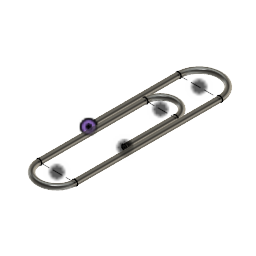
Day3Paperclip (Autodesk Fusion 360 design; units mm, degrees)
part number: 2025-11-19-20-14-40-836
Autodesk Fusion 360 part; units mm, degrees
sketch "Sweep" plane through (0, 0, 0) normal (0, 0, 1) x (1, 0, 0)
  line L0 (0, 0) -> (0, 16.25)
  line L1 (0, 16.25) -> (7.5, 16.25) construction
  line L2 (7.5, 16.25) -> (7.5, -10)
  line L3 (1, -10) -> (1, 9.25)
  line L4 (7.5, -10) -> (1, -10) construction
  line L5 (1, 9.25) -> (6.5, 9.25) construction
  line L6 (6.5, 9.25) -> (6.5, 0)
  arc A0 (7.5, 16.25) -> (0, 16.25) centre (3.75, 16.25) ccw
  arc A1 (6.5, 9.25) -> (1, 9.25) centre (3.75, 9.25) ccw
  arc A2 (1, -10) -> (7.5, -10) centre (4.25, -10) ccw
  dimension "d1" = 16.25
  dimension "d2" = 7.5
  dimension "d4" = 19.25
  dimension "d5" = 5.5
  dimension "d6" = 26.25
  dimension "d7" = 6.5
  dimension "d8" = 9.25
  constraint coincident L0.start origin
  constraint vertical L0
  constraint perpendicular L0 L1
  constraint perpendicular L1 L2
  constraint perpendicular L3 L4
  constraint perpendicular L3 L5
  constraint perpendicular L4 L6
  constraint vertical L3
  constraint tangent L0 A0
  constraint tangent L3 A1
  constraint tangent L3 A2
  measures "d1" distance of L0.start L0.end
  measures "d2" distance of L0.end L1.end
  measures "d4" distance of L3.start L3.end
  measures "d5" distance of L3.end L5.end
  measures "d6" distance of L1.end L2.end
  measures "d7" distance of L2.end L3.start
  measures "d8" distance of L5.end L6.end
sketch "Sketch2" plane through (0, 0, 0) normal (0, 1, 0) x (1, 0, 0)
  circle A0 centre (0, 0) radius 0.5
  dimension "d9" = 1
  constraint coincident A0.centre origin
  measures "d9" diameter of A0
sweep "Sweep1" add profiles "Sketch2" path "Sweep" along L0 A0 L2 A2 L3 A1 L6 section 1
